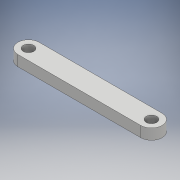
# Autodesk Inventor part: panto_linkageB
Saved by Autodesk Inventor 2017 (Build 210142000, 142)
## iProperties
Created: 2018-01-12
Part Number: panto_linkageB
Material: Generic
Document SubType Name: Modeling
Designer: Nic
Density: 1 g/cm^3
Appearance: Default
Author: Nic
Autodesk Inventor part; units mm, degrees
ref_plane "YZ Plane" through (0, 0, 0) normal (1, 0, 0) x (0, 1, 0)
ref_plane "XZ Plane" through (0, 0, 0) normal (0, 1, 0) x (-1, 0, 0)
ref_plane "XY Plane" through (0, 0, 0) normal (0, 0, 1) x (1, 0, 0)
sketch "Sketch1" plane through (0, 0, 0) normal (0, 0, 1) x (1, 0, 0)
  circle A0 centre (0, 0) radius 1
  circle A1 centre (-23.2, 0) radius 1
  line L0 (-23.2, 2) -> (0, 2)
  arc A2 (0, -2) -> (0, 2) centre (0, 0) ccw
  line L1 (0, -2) -> (-23.2, -2)
  arc A3 (-23.2, 2) -> (-23.2, -2) centre (-23.2, 0) ccw
  dimension "d0" = 2
  dimension "d1" = 23.2
  dimension "d2" = 2
  constraints: 4 centre point, 4 end point, 4 point on circle, 4 tangent, 2 vertical alignment, 1 coincident, 1 concentric, 1 equal radius, 1 horizontal, 1 horizontal alignment, 1 parallel
  measures "d0" diameter of A0
  measures "d1" distance of point (0, 0) A1.centre
  measures "d2" radius of A2
extrude "Extrusion1" add sketch "Sketch1" along normal blind 2
body "Solid1"
